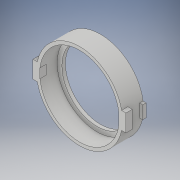
# Autodesk Inventor part: GelCupHolderTop
Saved by Autodesk Inventor 2018 (Build 220112000, 112)
## iProperties
Created: 2018-07-09
Part Number: GelCupHolderTop
Material: Generic
Document SubType Name: Modeling
Designer: brend
Density: 1 g/cm^3
Appearance: Default
Author: brend
Autodesk Inventor part; units mm, degrees
ref_plane "YZ Plane" through (0, 0, 0) normal (1, 0, 0) x (0, 1, 0)
ref_plane "XZ Plane" through (0, 0, 0) normal (0, 1, 0) x (-1, 0, 0)
ref_plane "XY Plane" through (0, 0, 0) normal (0, 0, 1) x (1, 0, 0)
sketch "Sketch1" plane through (0, 0, 0) normal (0, 0, 1) x (1, 0, 0)
  circle A0 centre (0, 0) radius 15.5575
  dimension "d0" = 31.115
  constraints: 1 centre point, 1 coincident
  measures "d0" diameter of A0
extrude "Extrusion1" add sketch "Sketch1" along normal blind 7.62
sketch "Sketch2" plane through (0, 0, 7.62) normal (0, 0, 1) x (1, 0, 0)
  circle A0 centre (0, 0) radius 14.3891
  dimension "d16" = 28.7782
  constraints: 1 centre point, 1 coincident
  measures "d16" diameter of A0
extrude "Extrusion2" cut sketch "Sketch2" against normal blind 6.35
sketch "Sketch3" plane through (0, 0, 0) normal (0, 0, -1) x (-1, 0, 0)
  circle A0 centre (0, 0) radius 12.7
  dimension "d15" = 25.4
  constraints: 1 centre point, 1 coincident
  measures "d15" diameter of A0
extrude "Extrusion3" cut sketch "Sketch3" against normal blind 5.08
sketch "Sketch4" plane through (0, 0, 7.62) normal (0, 0, 1) x (1, 0, 0)
  line L0 (-14.2875, -3.1369) -> (-16.8275, -3.1369)
  line L1 (-16.8275, -3.1369) -> (-16.8275, 3.1369)
  line L2 (-16.8275, 3.1369) -> (-14.2875, 3.1369)
  line L3 (-14.2875, 3.1369) -> (-14.2875, -3.1369)
  circle A0 centre (0, 0) radius 15.5575 projected
  line L4 (-14.2875, -3.1369) -> (-16.8275, 3.1369) construction
  line L5 (-16.8275, -3.1369) -> (-14.2875, 3.1369) construction
  line L6 (14.2875, -3.1369) -> (16.8275, -3.1369)
  line L7 (16.8275, -3.1369) -> (16.8275, 3.1369)
  line L8 (16.8275, 3.1369) -> (14.2875, 3.1369)
  line L9 (14.2875, 3.1369) -> (14.2875, -3.1369)
  line L10 (14.2875, -3.1369) -> (16.8275, 3.1369) construction
  line L11 (16.8275, -3.1369) -> (14.2875, 3.1369) construction
  point P0 (-15.5575, 0)
  point P1 (15.5575, 0)
  dimension "d7" = 2.54
  dimension "d8" = 6.2738
  dimension "d9" = 2.54
  dimension "d10" = 6.2738
  constraints: 24 end point, 4 midpoint, 4 parallel, 2 horizontal, 2 perpendicular, 2 point on circle
  measures "d7" distance of L1.end L2.end
  measures "d8" distance of L0.end L1.end
  measures "d9" distance of L8.end L7.end
  measures "d10" distance of L7.end L6.end
extrude "Extrusion5" add sketch "Sketch4" against normal blind 2.286 contours L0 A0 L2 L3 | L0 L1 L2 A0 | L6 L9 L8 A0 | A0 L8 L7 L6
sketch "Sketch5" plane through (0, 0, 0) normal (0, 0, -1) x (-1, 0, 0)
  line L0 (13.97, 2.3319) -> (16.51, 2.3319)
  line L1 (16.51, 2.3319) -> (16.51, -2.3319)
  line L2 (16.51, -2.3319) -> (13.97, -2.3319)
  line L3 (13.97, -2.3319) -> (13.97, 2.3319)
  line L4 (13.97, 2.3319) -> (16.51, -2.3319) construction
  line L5 (16.51, 2.3319) -> (13.97, -2.3319) construction
  line L6 (-16.51, 2.3319) -> (-13.97, 2.3319)
  line L7 (-13.97, 2.3319) -> (-13.97, -2.3319)
  line L8 (-13.97, -2.3319) -> (-16.51, -2.3319)
  line L9 (-16.51, -2.3319) -> (-16.51, 2.3319)
  line L10 (-16.51, 2.3319) -> (-13.97, -2.3319) construction
  line L11 (-13.97, 2.3319) -> (-16.51, -2.3319) construction
  point P0 (0, 0)
  point P1 (15.24, 0)
  point P2 (-15.24, 0)
  dimension "d17" = 2.54
  dimension "d18" = 2.54
  dimension "d19" = 15.24
  dimension "d20" = 15.24
  constraints: 24 end point, 4 midpoint, 4 parallel, 2 horizontal, 2 perpendicular, 1 point on line
  measures "d17" distance of L1.end L2.end
  measures "d18" distance of L7.end L8.end
  measures "d19" distance of point (0, 0) point (15.24, 0)
  measures "d20" distance of point (0, 0) point (-15.24, 0)
extrude "Extrusion6" add sketch "Sketch5" against normal blind 1.27
equation "\"d20\" = d19"
body "Solid1"
